ansi41sprocket1006 (Autodesk Fusion 360 design; units mm, degrees)
Autodesk Fusion 360 part; units mm, degrees
note: some values were not read from the file. Set by a fixed rule: which sketch regions a step uses.
sketch "Sketch1" plane through (0, 0, 0) normal (0, 0, 1) x (1, 0, 0)
  line L0 (-2.8829, 0) -> (0, 0)
  line L1 (-2.8829, 0) -> (-2.8829, 17.018)
  line L2 (-2.8829, 17.018) -> (-1.2954, 23.368)
  line L3 (-1.2954, 23.368) -> (0, 23.368)
  line L4 (0, 150) -> (0, -70) construction
  line L5 (-20.32, 10.2745) -> (20.32, 10.2745) construction
  line L6 (2.8829, 0) -> (2.8829, 17.018)
  line L7 (2.8829, 0) -> (-2.8829, 0)
  line L8 (2.8829, 17.018) -> (1.2954, 23.368)
  line L9 (1.2954, 23.368) -> (0, 23.368)
  line L10 (2.8829, 0) -> (-19.3421, 0) construction
  dimension "d7" = 6.35
  dimension "d8" = 1.5875
  dimension "d10" = 5.7658
  dimension "d11" = 22.225
  dimension "d12" = 23.368
  dimension "d56" = 10.2745
  measures "d7" distance of L1.end L3
  measures "d8" distance of L1.end L2.end
  measures "d10" distance of L1 L6
  measures "d11" distance of L6.start L10.end
  measures "d12" distance of L9 L10
  measures "d18" distance of L1.end
  measures "d25" distance of L1.end
  measures "d31" distance of L1.end
  measures "d56" distance of L5 L10
sketch "Sketch2" plane through (0, 0, 0) normal (1, 0, 0) x (0, 0, -1)
  circle A0 centre (0, 0) radius 20.549 construction
  circle A1 centre (0, 0) radius 21.606 construction
  circle A2 centre (0, 0) radius 29.9909 construction
  line L0 (0, 0) -> (20.549, 0) construction
  line L1 (20.549, 0) -> (10.2745, -17.796) construction
  line L2 (0, 0) -> (10.2745, -17.796) construction
  circle A3 centre (10.2745, -17.796) radius 3.8862 construction
  circle A4 centre (10.2745, -17.796) radius 3.9262 construction
  line L3 (0, 27.94) -> (0, -29.9909) construction
  line L4 (1.188, -23.0421) -> (12.8259, -16.3229) construction
  arc A5 (11.5528, -14.0836) -> (8.3114, -14.3958) centre (10.2745, -17.796) ccw
  line L5 (10.2745, -17.796) -> (-11.7452, -17.796) construction
  line L6 (-11.8689, -21.606) -> (10.16, -21.606) construction
  line L7 (11.5528, -14.0836) -> (0, -47.6354) construction
  arc A6 (8.3114, -14.3958) -> (6.4204, -17.0468) centre (10.2745, -17.796) ccw
  circle A7 centre (10.2745, -17.796) radius 3.8862 construction
  line L8 (0, -9.3854) -> (7.1033, -21.6888) construction
  line L9 (49.2566, 0) -> (7.0937, -24.3428) construction
  line L10 (8.2502, -23.6751) -> (22.7015, 0) construction
  arc A8 (13.5354, -15.0166) -> (11.5528, -14.0836) centre (8.2502, -23.6751) ccw
  line L11 (13.5354, -15.0166) -> (23.9626, -21.3814) construction
  line L12 (15.7152, -8.3724) -> (222.7749, -142.7367)
  line L13 (13.5354, -15.0166) -> (222.7749, -142.7367)
  point P0 (15.7152, -8.3724)
  point P1 (-0.6068, -17.796)
  dimension "d13" = 20.549
  dimension "d15" = 7.7724
  dimension "d16" = 7.8525
  dimension "d17" = 3.9262
  dimension "d18" = 3.81
  dimension "d23" = 10.8814
  dimension "d24" = 41
  dimension "d25" = 4.6927
  dimension "d26" = 4.0793
  dimension "d27" = 12.4
  measures "d13" distance of L0.end L1.end
  measures "d15" diameter of A3
  measures "d16" diameter of A4
  measures "d17" radius of A5
  measures "d18" distance of L5 L6
  measures "d23" distance of L1.end P0
  measures "d24" angle of L4 L7
  measures "d25" distance of L2 L8
  measures "d26" distance of L4 L9
  measures "d27" angle of L7 L10
sketch "Sketch3" plane through (0, 0, 0) normal (1, 0, 0) x (0, 0, -1)
  circle A0 centre (0, 0) radius 20.549 construction
  circle A1 centre (0, 0) radius 24.359 construction
  circle A2 centre (4.4103, -20.0702) radius 3.9437 construction
  circle A3 centre (4.4103, -20.0702) radius 3.8862 construction
  line L0 (4.4103, -20.0702) -> (15.365, -13.6448) construction
  line L1 (-18.0844, 61.7025) -> (15.365, -13.6448) construction
  line L2 (0, 0) -> (4.5156, -20.549) construction
  line L3 (-1.0511, -17.0815) -> (0.7025, -25.0616) construction
  line L4 (0, 0) -> (0, -85.9346) construction
  line L5 (11.1742, -18.5838) -> (-367394.3879, -80754.4852) construction
  line L6 (0.7025, -25.0616) -> (47.7422, -14.7248) construction
  line L7 (0.7025, -25.0616) -> (1.0731, -24.5626) construction
  arc A4 (8.3723, -18.3958) -> (6.762, -16.9043) centre (0.7025, -25.0616) ccw
  line L8 (0.7025, -25.0616) -> (100.5359, 61.7025) construction
  line L9 (25.3874, -67.3127) -> (13.7963, -14.5649) construction
  line L10 (13.7963, -14.5649) -> (52.2114, -6.1233) construction
  line L11 (8.3723, -18.3958) -> (8.8095, -18.8988)
  line L12 (13.7963, -14.5649) -> (8.8095, -18.8988) construction
  line L13 (0.1114, -20.2111) -> (-0.0746, -20.8511)
  arc A5 (0.948, -18.1819) -> (0.1114, -20.2111) centre (9.8692, -23.0473) ccw
  line L14 (-35.56, -20.549) -> (40.64, -20.549) construction
  line L15 (-43.18, -24.359) -> (38.1, -24.359) construction
  arc A6 (6.762, -16.9043) -> (0.948, -18.1819) centre (4.4103, -20.0702) ccw
  arc A7 (8.8095, -18.8988) -> (12.3203, -21.0048) centre (13.7963, -14.5649) ccw
  line L16 (0, 0) -> (12.3241, -21.0114) construction
  line L17 (13.1016, -22.3369) -> (59.9065, -102.1346) construction
  arc A8 (-2.379, -24.2349) -> (-0.0746, -20.8511) centre (-6.419, -19.0071) ccw
  arc A9 (12.3203, -21.0048) -> (12.1956, -16.9127) centre (5.979, -19.1501) ccw
  line L18 (11.9699, -16.2857) -> (12.1956, -16.9127)
  arc A10 (11.454, -14.1523) -> (11.9699, -16.2857) centre (21.5312, -12.8446) ccw
  arc A11 (15.4067, -9.7013) -> (11.454, -14.1523) centre (15.365, -13.6448) ccw
  arc A12 (17.5862, -9.9614) -> (15.4067, -9.7013) centre (15.2992, -19.8623) ccw
  line L19 (17.5862, -9.9614) -> (18.2355, -10.1114)
  arc A13 (18.2355, -10.1114) -> (22.3136, -9.7516) centre (19.7225, -3.674) ccw
  arc A14 (22.3136, -9.7516) -> (19.8075, -6.5143) centre (16.0933, -11.9783) ccw
  line L20 (19.2564, -6.1397) -> (19.8075, -6.5143)
  arc A15 (17.585, -4.7169) -> (19.2564, -6.1397) centre (24.969, 2.2642) ccw
  arc A16 (18.1666, 1.2074) -> (17.585, -4.7169) centre (20.4507, -2.0075) ccw
  arc A17 (20.0827, 2.2779) -> (18.1666, 1.2074) centre (24.0521, -7.0763) ccw
  line L21 (20.0827, 2.2779) -> (20.6962, 2.5383)
  arc A18 (20.6962, 2.5383) -> (23.7839, 5.2264) centre (18.1153, 8.6202) ccw
  arc A19 (23.7839, 5.2264) -> (19.8536, 6.3724) centre (20.0604, -0.2313) ccw
  line L22 (19.1875, 6.3515) -> (19.8536, 6.3724)
  arc A20 (16.9991, 6.5202) -> (19.1875, 6.3515) centre (18.8695, 16.5082) ccw
  arc A21 (13.9874, 11.6548) -> (16.9991, 6.5202) centre (17.725, 10.3965) ccw
  arc A22 (14.9083, 13.6472) -> (13.9874, 11.6548) centre (23.6179, 8.4126) ccw
  line L23 (14.9083, 13.6472) -> (15.2516, 14.2184)
  arc A23 (15.2516, 14.2184) -> (16.1696, 18.2081) centre (9.5887, 17.6218) ccw
  arc A24 (16.1696, 18.2081) -> (12.3163, 16.825) centre (16.3652, 11.6041) ccw
  line L24 (11.7897, 16.4166) -> (12.3163, 16.825)
  arc A25 (9.9201, 15.2667) -> (11.7897, 16.4166) centre (5.5625, 24.4466) ccw
  arc A26 (4.4655, 17.6505) -> (9.9201, 15.2667) centre (8.2289, 18.8294) ccw
  arc A27 (4.0394, 19.8037) -> (4.4655, 17.6505) centre (14.1625, 20.6882) ccw
  line L25 (4.0394, 19.8037) -> (3.9814, 20.4676)
  arc A28 (3.9814, 20.4676) -> (2.379, 24.2349) centre (-2.6004, 19.8925) ccw
  arc A29 (2.379, 24.2349) -> (0.0746, 20.8511) centre (6.419, 19.0071) ccw
  line L26 (-0.1114, 20.2111) -> (0.0746, 20.8511)
  arc A30 (-0.948, 18.1819) -> (-0.1114, 20.2111) centre (-9.8692, 23.0473) ccw
  arc A31 (-6.762, 16.9043) -> (-0.948, 18.1819) centre (-4.4103, 20.0702) ccw
  arc A32 (-8.3723, 18.3958) -> (-6.762, 16.9043) centre (-0.7025, 25.0616) ccw
  line L27 (-8.3723, 18.3958) -> (-8.8095, 18.8988)
  arc A33 (-8.8095, 18.8988) -> (-12.3203, 21.0048) centre (-13.7963, 14.5649) ccw
  circle A34 centre (0, 0) radius 24.3514
  arc A35 (-12.3203, 21.0048) -> (-12.1956, 16.9127) centre (-5.979, 19.1501) ccw
  line L28 (-11.9699, 16.2857) -> (-12.1956, 16.9127)
  arc A36 (-11.454, 14.1523) -> (-11.9699, 16.2857) centre (-21.5312, 12.8446) ccw
  arc A37 (-15.4067, 9.7013) -> (-11.454, 14.1523) centre (-15.365, 13.6448) ccw
  arc A38 (-17.5862, 9.9614) -> (-15.4067, 9.7013) centre (-15.2992, 19.8623) ccw
  line L29 (-17.5862, 9.9614) -> (-18.2355, 10.1114)
  arc A39 (-18.2355, 10.1114) -> (-22.3136, 9.7516) centre (-19.7225, 3.674) ccw
  arc A40 (-22.3136, 9.7516) -> (-19.8075, 6.5143) centre (-16.0933, 11.9783) ccw
  line L30 (-19.2564, 6.1397) -> (-19.8075, 6.5143)
  arc A41 (-17.585, 4.7169) -> (-19.2564, 6.1397) centre (-24.969, -2.2642) ccw
  arc A42 (-18.1666, -1.2074) -> (-17.585, 4.7169) centre (-20.4507, 2.0075) ccw
  arc A43 (-20.0827, -2.2779) -> (-18.1666, -1.2074) centre (-24.0521, 7.0763) ccw
  line L31 (-20.0827, -2.2779) -> (-20.6962, -2.5383)
  arc A44 (-20.6962, -2.5383) -> (-23.7839, -5.2264) centre (-18.1153, -8.6202) ccw
  arc A45 (-23.7839, -5.2264) -> (-19.8536, -6.3724) centre (-20.0604, 0.2313) ccw
  line L32 (-19.1875, -6.3515) -> (-19.8536, -6.3724)
  arc A46 (-16.9991, -6.5202) -> (-19.1875, -6.3515) centre (-18.8695, -16.5082) ccw
  arc A47 (-13.9874, -11.6548) -> (-16.9991, -6.5202) centre (-17.725, -10.3965) ccw
  arc A48 (-14.9083, -13.6472) -> (-13.9874, -11.6548) centre (-23.6179, -8.4126) ccw
  line L33 (-14.9083, -13.6472) -> (-15.2516, -14.2184)
  arc A49 (-15.2516, -14.2184) -> (-16.1696, -18.2081) centre (-9.5887, -17.6218) ccw
  arc A50 (-16.1696, -18.2081) -> (-12.3163, -16.825) centre (-16.3652, -11.6041) ccw
  line L34 (-11.7897, -16.4166) -> (-12.3163, -16.825)
  arc A51 (-9.9201, -15.2667) -> (-11.7897, -16.4166) centre (-5.5625, -24.4466) ccw
  arc A52 (-4.4655, -17.6505) -> (-9.9201, -15.2667) centre (-8.2289, -18.8294) ccw
  arc A53 (-4.0394, -19.8037) -> (-4.4655, -17.6505) centre (-14.1625, -20.6882) ccw
  line L35 (-4.0394, -19.8037) -> (-3.9814, -20.4676)
  arc A54 (-3.9814, -20.4676) -> (-2.379, -24.2349) centre (2.6004, -19.8925) ccw
  point P0 (-6.419, -19.0071)
  dimension "d28" = 7.7724
  dimension "d29" = 7.8875
  dimension "d30" = 12.7
  dimension "d31" = 4.6927
  dimension "d37" = 4.0793
  dimension "d38" = 36.5
  dimension "d39" = 12.4
  dimension "d40" = 10.3488
  dimension "d41" = 3.3625
  dimension "d42" = 3.81
  dimension "d43" = 3.9437
  dimension "d45" = 18
  dimension "d47" = 360
  measures "d28" diameter of A3
  measures "d29" diameter of A2
  measures "d30" distance of A2.centre L0.end
  measures "d31" distance of L2 L3
  measures "d37" distance of L5 L6
  measures "d39" angle of L7 L8
  measures "d40" distance of L2 L9
  measures "d41" distance of L5 L10
  measures "d42" distance of L14 L15
  measures "d43" radius of A6
  measures "d45" angle of L2 L16
revolve "Revolve1" add sketch "Sketch1" angle 360 about axis through (2.8829, 0, 0) along (-1, 0, 0)
extrude "Extrude1" cut sketch "Sketch3" along normal mid plane 10.16 contours A4 L11 L13 A5 A6 A7 A8 A34
pattern_circular "C-Pattern1" count 10 over 360 about axis through (2.8829, 0, 0) along (-1, 0, 0) of "Extrude1"
sketch "Sketch4" plane through (-2.8829, 0, 0) normal (-1, 0, 0) x (0, 0, 1)
  circle A0 centre (0, 0) radius 15.875
  arc A1 (-11.6085, -12.4441) -> (-13.7288, -10.0565) centre (-15.365, -13.6448) ccw
  arc A2 (-11.6085, -12.4441) -> (-5.1958, -16.2054) centre (0, 0) ccw
  arc A3 (-2.077, -16.8908) -> (-5.1958, -16.2054) centre (-4.4103, -20.0702) ccw
  arc A4 (-2.077, -16.8908) -> (5.3219, -16.1645) centre (0, 0) ccw
  arc A5 (8.2478, -14.8858) -> (5.3219, -16.1645) centre (8.2289, -18.8294) ccw
  arc A6 (8.2478, -14.8858) -> (13.8067, -9.9492) centre (0, 0) ccw
  arc A7 (15.4223, -7.1949) -> (13.8067, -9.9492) centre (17.725, -10.3965) ccw
  arc A8 (15.4223, -7.1949) -> (17.0179, 0.0663) centre (0, 0) ccw
  arc A9 (16.7059, 3.2442) -> (17.0179, 0.0663) centre (20.4507, 2.0075) ccw
  arc A10 (16.7059, 3.2442) -> (13.7288, 10.0565) centre (0, 0) ccw
  arc A11 (11.6085, 12.4441) -> (13.7288, 10.0565) centre (15.365, 13.6448) ccw
  arc A12 (11.6085, 12.4441) -> (5.1958, 16.2054) centre (0, 0) ccw
  arc A13 (2.077, 16.8908) -> (5.1958, 16.2054) centre (4.4103, 20.0702) ccw
  arc A14 (2.077, 16.8908) -> (-5.3219, 16.1645) centre (0, 0) ccw
  arc A15 (-8.2478, 14.8858) -> (-5.3219, 16.1645) centre (-8.2289, 18.8294) ccw
  arc A16 (-8.2478, 14.8858) -> (-13.8067, 9.9492) centre (0, 0) ccw
  arc A17 (-15.4223, 7.1949) -> (-13.8067, 9.9492) centre (-17.725, 10.3965) ccw
  arc A18 (-15.4223, 7.1949) -> (-17.0179, -0.0663) centre (0, 0) ccw
  arc A19 (-16.7059, -3.2442) -> (-17.0179, -0.0663) centre (-20.4507, -2.0075) ccw
  arc A20 (-16.7059, -3.2442) -> (-13.7288, -10.0565) centre (0, 0) ccw
  dimension "d53" = 31.75
  measures "d53" diameter of A0
extrude "Extrude2" add sketch "Sketch4" along normal up to surface (16.4592 mm away) contours A0
sketch "Sketch5" plane through (0, 0, 0) normal (0, 0, 1) x (1, 0, 0)
  line L0 (-2.8829, 18.415) -> (-2.8829, 10.2745)
  line L1 (-2.8829, 10.2745) -> (-6.4865, 10.2745)
  line L2 (-6.4865, 10.2745) -> (-6.4865, 18.415)
  line L3 (-6.4865, 18.415) -> (-2.8829, 18.415)
  line L4 (-20.32, 10.2745) -> (20.32, 10.2745)
  line L5 (2.8829, 0) -> (-19.3421, 0)
  line L6 (-18.7071, 15.875) -> (-19.3421, 15.875)
  line L7 (-19.3421, 15.875) -> (-19.3421, 15.24)
  line L8 (-19.3421, 15.24) -> (-18.7071, 15.875)
  line L9 (-2.8829, -14.8858) -> (-2.8829, -9.9492)
  line L10 (-2.8829, 3.2442) -> (-2.8829, 10.0565)
  line L11 (-2.8829, 9.9492) -> (-2.8829, 14.8858)
  line L12 (-2.8829, 12.4441) -> (-2.8829, 16.2054)
  line L13 (-2.8829, -10.0565) -> (-2.8829, -3.2442)
  point P0 (-19.3421, 0)
  dimension "d57" = 18.415
  dimension "d58" = 3.6036
  dimension "d59" = 15.875
  dimension "d60" = 0.635
  measures "d57" distance of L3 L5
  measures "d58" distance of L0.start L2.end
  measures "d59" distance of L6 P0
  measures "d60" distance of L6.start L6.end
revolve "Revolve2" cut sketch "Sketch5" angle 360 about axis through (2.8829, 0, 0) along (-1, 0, 0)
sketch "Sketch6" plane through (2.8829, 0, 0) normal (1, 0, 0) x (0, 0, -1)
  circle A0 centre (0, 0) radius 7.9375
  arc A1 (13.7288, -10.0565) -> (11.6085, -12.4441) centre (15.365, -13.6448) ccw
  arc A2 (13.7288, -10.0565) -> (16.7059, -3.2442) centre (0, 0) ccw
  arc A3 (17.0179, -0.0663) -> (16.7059, -3.2442) centre (20.4507, -2.0075) ccw
  arc A4 (17.0179, -0.0663) -> (15.4223, 7.1949) centre (0, 0) ccw
  arc A5 (13.8067, 9.9492) -> (15.4223, 7.1949) centre (17.725, 10.3965) ccw
  arc A6 (13.8067, 9.9492) -> (8.2478, 14.8858) centre (0, 0) ccw
  arc A7 (5.3219, 16.1645) -> (8.2478, 14.8858) centre (8.2289, 18.8294) ccw
  arc A8 (5.3219, 16.1645) -> (-2.077, 16.8908) centre (0, 0) ccw
  arc A9 (-5.1958, 16.2054) -> (-2.077, 16.8908) centre (-4.4103, 20.0702) ccw
  arc A10 (-5.1958, 16.2054) -> (-11.6085, 12.4441) centre (0, 0) ccw
  arc A11 (-13.7288, 10.0565) -> (-11.6085, 12.4441) centre (-15.365, 13.6448) ccw
  arc A12 (-13.7288, 10.0565) -> (-16.7059, 3.2442) centre (0, 0) ccw
  arc A13 (-17.0179, 0.0663) -> (-16.7059, 3.2442) centre (-20.4507, 2.0075) ccw
  arc A14 (-17.0179, 0.0663) -> (-15.4223, -7.1949) centre (0, 0) ccw
  arc A15 (-13.8067, -9.9492) -> (-15.4223, -7.1949) centre (-17.725, -10.3965) ccw
  arc A16 (-13.8067, -9.9492) -> (-8.2478, -14.8858) centre (0, 0) ccw
  arc A17 (-5.3219, -16.1645) -> (-8.2478, -14.8858) centre (-8.2289, -18.8294) ccw
  arc A18 (-5.3219, -16.1645) -> (2.077, -16.8908) centre (0, 0) ccw
  arc A19 (5.1958, -16.2054) -> (2.077, -16.8908) centre (4.4103, -20.0702) ccw
  arc A20 (5.1958, -16.2054) -> (11.6085, -12.4441) centre (0, 0) ccw
  dimension "d62" = 15.875
  measures "d62" diameter of A0
extrude "Extrude3" cut sketch "Sketch6" against normal up to surface (22.225 mm away) contours A0
equation "No_teeth = 10"
equation "Innershaft_dia = ( 5 / 8 ) * 1 in"
equation "OD = 1.84 in"
equation "Overall_width = ( 7 / 8 ) * 1 in"
equation "Hub_dia = 1 1/4\""
equation "Gear_thickness = 0.227 in"
equation "d7 = Tooth_pitch / 2"
equation "d8 = d7 / 4"
equation "d10 = Gear_thickness"
equation "d11 = Overall_width"
equation "d12 = OD / 2"
equation "d13 = Tooth_pitch / sin(( 180 / No_teeth ) * 1 deg) / 2"
equation "Tooth_pitch = 0.5 in"
equation "d16 = 1.0005 * d15 + 0.003 in"
equation "d17 = d16 / 2"
equation "d23 = 1.4 * d15"
equation "d24 = 35 deg + ( ( 60 / No_teeth ) * 1 deg )"
equation "d25 = 0.8 * d15 * cos(35 deg + ( ( 60 / No_teeth ) * 1 deg ))"
equation "d26 = 0.8 * d15 * sin(35 deg + ( ( 60 / No_teeth ) * 1 deg ))"
equation "d27 = 18 deg - ( ( 56 / No_teeth ) * 1 deg )"
equation "d29 = 1.005 * d28 + 0.003 in"
equation "d30 = Tooth_pitch"
equation "d31 = 0.8 * d28 * cos(35 deg + ( ( 60 / No_teeth ) * 1 deg ))"
equation "d37 = 0.8 * d28 * sin(35 deg + ( ( 60 / No_teeth ) * 1 deg ))"
equation "d39 = 18 deg - ( ( 56 / No_teeth ) * 1 deg )"
equation "d40 = 1.4 * d28 * cos(( 180 / No_teeth ) * 1 deg)"
equation "d41 = 1.4 * d28 * sin(( 180 / No_teeth ) * 1 deg)"
equation "d42 = 0.3 * d30"
equation "d43 = d29 / 2"
equation "d45 = ( 180 / No_teeth ) * 1 deg"
equation "d46 = No_teeth"
equation "d51 = No_teeth"
equation "d53 = Hub_dia"
equation "d56 = pitch_cir_dia / 4"
equation "d57 = Hub_dia / 2 + 0.1 in"
equation "d58 = Gear_thickness * 5 / 8"
equation "d59 = Hub_dia / 2"
equation "d62 = Innershaft_dia"
equation "pitch_cir_dia = ( 0.5 / sin(( 180 / No_teeth ) * 1 deg) ) * 1 in"
